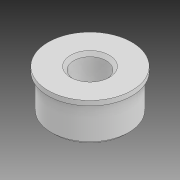
# Autodesk Inventor part: ShaftSpacer
Saved by Autodesk Inventor 2020 (Build 240168000, 168)
## iProperties
Created: 2021-10-30
Part Number: ShaftSpacer
Material: Generic
Document SubType Name: Modeling
Designer: DDeGo
Density: 1 g/cm^3
Appearance: Default
Author: DDeGo
Autodesk Inventor part; units mm, degrees
ref_plane "YZ Plane" through (0, 0, 0) normal (1, 0, 0) x (0, 1, 0)
ref_plane "XZ Plane" through (0, 0, 0) normal (0, 1, 0) x (-1, 0, 0)
ref_plane "XY Plane" through (0, 0, 0) normal (0, 0, 1) x (1, 0, 0)
sketch "Sketch1" plane through (0, 0, 0) normal (0, 0, 1) x (1, 0, 0)
  line L0 (0, 2.6) -> (0, 0.3) construction
  line L1 (0, 0) -> (1.025, 0)
  line L2 (1.025, 2.6) -> (0, 2.6) construction
  line L3 (1.025, 2.6) -> (2.65, 2.6)
  line L4 (2.65, 2.6) -> (2.65, 2.3)
  line L5 (2.65, 2.3) -> (2.45, 2.3)
  line L6 (2.45, 2.3) -> (2.45, 0)
  line L7 (2.45, 0) -> (1.025, 0)
  line L8 (1.025, 2.6) -> (1.025, 0.3)
  line L9 (1.025, 0.3) -> (1.025, 0) construction
  line L10 (1.025, 0.3) -> (0, 0.3)
  line L11 (0, 0.3) -> (0, 0)
  dimension "d0" = 2.45
  dimension "d2" = 0.3
  dimension "d3" = 0.2
  dimension "d4" = 2.3
  dimension "d9" = 0.3
  dimension "d10" = 1.025
  constraints: 24 end point, 9 perpendicular, 3 vertical, 2 horizontal
  measures "d0" distance between parallel lines of L0 L6
  measures "d2" distance of L3.end L4.end
  measures "d3" distance of L4.end L5.end
  measures "d4" distance of L5.end L6.end
  measures "d9" distance between parallel lines of L1 L10
  measures "d10" distance between parallel lines of L0 L8
revolve "Revolution1" add sketch "Sketch1" angle 360 about axis through (0, 2.6, 0) along (0, -1, 0)
chamfer "Chamfer1" distance 0.2 angle 45 2 edges at (-1.025, 2.6, 0) (-2.45, 0, 0)
body "Solid1"
